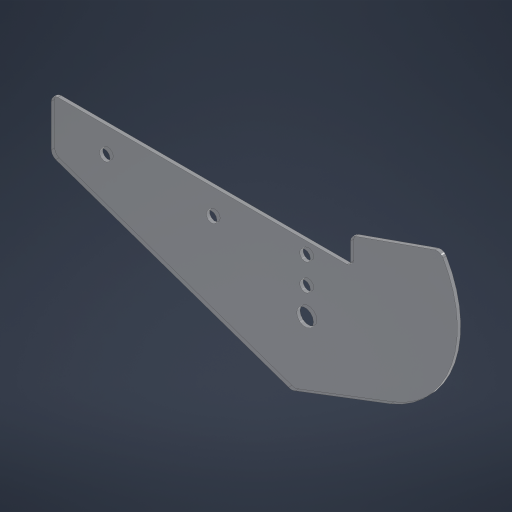
# Autodesk Inventor part: intake_sled
Saved by Autodesk Inventor 2024 (Build 280153000, 153)
## iProperties
Created: 2024-01-04
Part Number: intake_sled
Material: Generic
Document SubType Name: Modeling
Designer: macbook
Density: 1 g/cm^3
Appearance: Polycarbonate - Clear(1)
Author: macbook
Autodesk Inventor part; units mm, degrees
ref_plane "YZ Plane" through (0, 0, 0) normal (1, 0, 0) x (0, 1, 0)
ref_plane "XZ Plane" through (0, 0, 0) normal (0, 1, 0) x (-1, 0, 0)
ref_plane "XY Plane" through (0, 0, 0) normal (0, 0, 1) x (1, 0, 0)
sketch "Sketch1" plane through (0, 0, 0) normal (0, 0, 1) x (1, 0, 0)
  spline S0 degree 3 poles (57.6456, -40.773) (58.3081, -40.9936) (59.0965, -41.3227) (60.2711, -40.8533) (60.9829, -40.5929) knots 0 0 0 0 0.471955 1 1 1 1
  line L0 (57.6456, -40.773) -> (58.3081, -40.9936) construction
  line L1 (58.3081, -40.9936) -> (59.0965, -41.3227) construction
  line L2 (59.0965, -41.3227) -> (60.2711, -40.8533) construction
  line L3 (60.2711, -40.8533) -> (60.9829, -40.5929) construction
  circle A0 centre (65.4964, 17.3655) radius 2.54
  circle A1 centre (65.4964, 4.6655) radius 2.54
  circle A2 centre (65.4964, -8.0345) radius 4
  circle A3 centre (21.0464, 11.0155) radius 2.54
  arc A4 (106.077, -23.4013) -> (131.0436, 49.1793) centre (87.0864, 23.7155) ccw
  line L4 (87.0864, 25.303) -> (87.0864, 34.1689)
  line L5 (89.2051, 37.163) -> (127.2399, 50.5819)
  circle A5 centre (-29.7536, 11.0155) radius 2.54
  line L6 (-51.9786, 23.7155) -> (85.4989, 23.7155)
  line L7 (60.9829, -40.5929) -> (106.077, -23.4013)
  line L8 (-55.1536, 20.5405) -> (-55.1536, 0.5755)
  line L9 (-53.0182, -2.4244) -> (57.6456, -40.773)
  arc A6 (-51.9786, 23.7155) -> (-55.1536, 20.5405) centre (-51.9786, 20.5405) ccw
  arc A7 (-55.1536, 0.5755) -> (-53.0182, -2.4244) centre (-51.9786, 0.5755) ccw
  arc A8 (131.0436, 49.1793) -> (127.2399, 50.5819) centre (128.2963, 47.5878) ccw
  arc A9 (89.2051, 37.163) -> (87.0864, 34.1689) centre (90.2614, 34.1689) ccw
  arc A10 (85.4989, 23.7155) -> (87.0864, 25.303) centre (85.4989, 25.303) ccw
  point P0 (129.6573, 51.4348)
  point P1 (129.6573, 51.4348)
  point P2 (-55.1536, 23.7155)
  point P3 (-55.1536, -1.6845)
  point P4 (60.9902, -40.5901)
  point P5 (129.6573, 51.4348)
  point P6 (87.0864, 36.4155)
  point P7 (60.9829, -40.5929)
  dimension "d2" = 3.175
  dimension "d3" = 1.5875
  constraints: 13 point on circle, 12 end point, 11 centre point, 10 tangent, 3 equal radius, 1 point on line, 3 other
  measures "d2" radius of A6
  measures "d3" radius of A10
extrude "Extrusion1" add sketch "Sketch1" along normal blind 1.5875
body "Solid1"
